Autodesk Inventor part; units mm, degrees
(part 2 of 2)
  spline S27 degree 3 poles (53.2343, -1.5147) (53.2876, -1.6132) (53.3942, -1.8104) (53.5388, -2.114) (53.6487, -2.3717) (53.7287, -2.5811) (53.7846, -2.7396) (53.8352, -2.8999) (53.8989, -3.1148) (53.9296, -3.3095) (53.9849, -3.4685) (54.0166, -3.5312) (54.0472, -3.5782) (54.0738, -3.6107) (54.1026, -3.6414) (54.1344, -3.6689) (54.1689, -3.6931) (54.2057, -3.7134) (54.2441, -3.7308) (54.2847, -3.7418) (54.3257, -3.7514) (54.3818, -3.7547) (54.4518, -3.7553) (54.5217, -3.7582) (54.5779, -3.7578) (54.6193, -3.7503) (54.6605, -3.7414) (54.6997, -3.726) (54.7375, -3.7075) (54.7732, -3.6852) (54.8063, -3.6593) (54.8366, -3.6301) (54.8649, -3.599) (54.8979, -3.5536) (54.9327, -3.4926) (54.996, -3.3366) (55.0366, -3.1438) (55.1111, -2.9324) (55.1699, -2.7749) (55.2338, -2.6194) (55.3243, -2.4144) (55.4472, -2.1626) (55.607, -1.8667) (55.7235, -1.6753) (55.7818, -1.5795) knots 0 0 0 0 0.033613 0.067227 0.100839 0.117647 0.134454 0.151261 0.168068 0.201677 0.210077 0.218473 0.222676 0.226878 0.231076 0.235279 0.239479 0.24368 0.247882 0.252083 0.256283 0.260485 0.268889 0.277292 0.281494 0.285694 0.289895 0.294097 0.298298 0.302498 0.306701 0.310899 0.315101 0.319304 0.3277 0.3361 0.369709 0.386516 0.403323 0.420131 0.436938 0.470551 0.504164 0.537777 0.537777 0.537777 0.537777 projected
  arc A27 (53.2343, -1.5147) -> (52.4787, -1.5579) centre (54, -21.5) ccw projected
  spline S28 degree 3 poles (49.9552, -1.9133) (50.024, -2.0017) (50.1616, -2.1786) (50.3542, -2.4543) (50.5051, -2.6904) (50.6184, -2.8838) (50.6997, -3.0309) (50.776, -3.1807) (50.8742, -3.3822) (50.9365, -3.5691) (51.0172, -3.7169) (51.0588, -3.7735) (51.0967, -3.8148) (51.1284, -3.8426) (51.1618, -3.8681) (51.1977, -3.89) (51.2357, -3.9081) (51.2753, -3.9222) (51.3161, -3.933) (51.358, -3.9371) (51.4, -3.9399) (51.4558, -3.9339) (51.525, -3.9229) (51.5944, -3.9143) (51.6498, -3.9047) (51.6894, -3.8904) (51.7285, -3.8749) (51.7647, -3.8533) (51.7989, -3.8288) (51.8304, -3.8009) (51.8588, -3.7699) (51.8839, -3.7362) (51.9067, -3.7008) (51.9317, -3.6506) (51.956, -3.5847) (51.9928, -3.4204) (52.0011, -3.2235) (52.0398, -3.0027) (52.0719, -2.8377) (52.1093, -2.6738) (52.1648, -2.4567) (52.2446, -2.1881) (52.3536, -1.87) (52.437, -1.662) (52.4787, -1.5579) knots 0 0 0 0 0.033613 0.067227 0.100839 0.117647 0.134454 0.151261 0.168068 0.201677 0.210077 0.218473 0.222676 0.226878 0.231076 0.235279 0.239479 0.24368 0.247882 0.252083 0.256283 0.260485 0.268889 0.277292 0.281494 0.285694 0.289895 0.294097 0.298298 0.302498 0.306701 0.310899 0.315101 0.319304 0.3277 0.3361 0.369709 0.386516 0.403323 0.420131 0.436938 0.470551 0.504164 0.537777 0.537777 0.537777 0.537777 projected
  arc A28 (49.9552, -1.9133) -> (49.2171, -2.0803) centre (54, -21.5) ccw projected
  spline S29 degree 3 poles (46.7865, -2.8462) (46.869, -2.9221) (47.0338, -3.0739) (47.2691, -3.3141) (47.4568, -3.5222) (47.6004, -3.6943) (47.7048, -3.8261) (47.8047, -3.9612) (47.9347, -4.1438) (48.027, -4.3179) (48.1309, -4.4504) (48.1812, -4.4994) (48.2254, -4.5339) (48.2612, -4.556) (48.2984, -4.5757) (48.3374, -4.5914) (48.3779, -4.603) (48.4193, -4.6104) (48.4612, -4.6144) (48.5032, -4.6115) (48.5451, -4.6073) (48.5992, -4.5922) (48.6656, -4.57) (48.7327, -4.5501) (48.7857, -4.5315) (48.8225, -4.5109) (48.8585, -4.4892) (48.8906, -4.4619) (48.9203, -4.4321) (48.9468, -4.3994) (48.9698, -4.3641) (48.989, -4.3267) (49.0056, -4.2881) (49.022, -4.2345) (49.0352, -4.1655) (49.0444, -3.9974) (49.0202, -3.8018) (49.022, -3.5776) (49.0264, -3.4096) (49.0364, -3.2418) (49.0554, -3.0185) (49.0899, -2.7404) (49.145, -2.4087) (49.1931, -2.1898) (49.2171, -2.0803) knots 0 0 0 0 0.033613 0.067227 0.100839 0.117647 0.134454 0.151261 0.168068 0.201677 0.210077 0.218473 0.222676 0.226878 0.231076 0.235279 0.239479 0.24368 0.247882 0.252083 0.256283 0.260485 0.268889 0.277292 0.281494 0.285694 0.289895 0.294097 0.298298 0.302498 0.306701 0.310899 0.315101 0.319304 0.3277 0.3361 0.369709 0.386516 0.403323 0.420131 0.436938 0.470551 0.504164 0.537777 0.537777 0.537777 0.537777 projected
  arc A29 (46.7865, -2.8462) -> (46.0859, -3.1324) centre (54, -21.5) ccw projected
  spline S30 degree 3 poles (43.8146, -4.2879) (43.9084, -4.3492) (44.096, -4.4718) (44.3676, -4.67) (44.587, -4.8444) (44.757, -4.9905) (44.8816, -5.1033) (45.0024, -5.2201) (45.1607, -5.3789) (45.2804, -5.5354) (45.4047, -5.6489) (45.4624, -5.689) (45.5117, -5.7157) (45.5506, -5.7317) (45.5905, -5.745) (45.6316, -5.7541) (45.6734, -5.7589) (45.7155, -5.7593) (45.7575, -5.7563) (45.7984, -5.7466) (45.8391, -5.7356) (45.89, -5.7117) (45.9518, -5.6789) (46.0147, -5.6483) (46.0639, -5.6212) (46.0968, -5.5948) (46.1287, -5.5675) (46.1559, -5.5352) (46.1803, -5.501) (46.2011, -5.4644) (46.2179, -5.4258) (46.2307, -5.3857) (46.2407, -5.3449) (46.2481, -5.2893) (46.2497, -5.2191) (46.2311, -5.0517) (46.1751, -4.8628) (46.14, -4.6414) (46.1167, -4.475) (46.0989, -4.3078) (46.0809, -4.0844) (46.0692, -3.8045) (46.0689, -3.4682) (46.0803, -3.2443) (46.0859, -3.1324) knots 0 0 0 0 0.033613 0.067227 0.100839 0.117647 0.134454 0.151261 0.168068 0.201677 0.210077 0.218473 0.222676 0.226878 0.231076 0.235279 0.239479 0.24368 0.247882 0.252083 0.256283 0.260485 0.268889 0.277292 0.281494 0.285694 0.289895 0.294097 0.298298 0.302498 0.306701 0.310899 0.315101 0.319304 0.3277 0.3361 0.369709 0.386516 0.403323 0.420131 0.436938 0.470551 0.504164 0.537777 0.537777 0.537777 0.537777 projected
  arc A30 (43.8146, -4.2879) -> (43.1707, -4.6856) centre (54, -21.5) ccw projected
  spline S31 degree 3 poles (41.1205, -6.1991) (41.2231, -6.2441) (41.4283, -6.3342) (41.7289, -6.485) (41.9739, -6.6209) (42.1656, -6.737) (42.3071, -6.8277) (42.4455, -6.9231) (42.6278, -7.0536) (42.7716, -7.1883) (42.9129, -7.2799) (42.9764, -7.3099) (43.0294, -7.3282) (43.0705, -7.3375) (43.112, -7.344) (43.154, -7.3462) (43.1961, -7.3441) (43.2376, -7.3375) (43.2786, -7.3277) (43.3174, -7.3114) (43.3556, -7.2938) (43.4019, -7.2619) (43.4575, -7.2194) (43.5145, -7.1788) (43.5586, -7.144) (43.5866, -7.1126) (43.6137, -7.0803) (43.6351, -7.0441) (43.6536, -7.0063) (43.668, -6.9667) (43.6783, -6.9259) (43.6843, -6.8843) (43.6875, -6.8424) (43.6856, -6.7863) (43.6757, -6.7168) (43.6298, -6.5548) (43.5434, -6.3777) (43.4723, -6.1651) (43.422, -6.0047) (43.3769, -5.8428) (43.3224, -5.6254) (43.2647, -5.3512) (43.2092, -5.0195) (43.1835, -4.7969) (43.1707, -4.6856) knots 0 0 0 0 0.033613 0.067227 0.100839 0.117647 0.134454 0.151261 0.168068 0.201677 0.210077 0.218473 0.222676 0.226878 0.231076 0.235279 0.239479 0.24368 0.247882 0.252083 0.256283 0.260485 0.268889 0.277292 0.281494 0.285694 0.289895 0.294097 0.298298 0.302498 0.306701 0.310899 0.315101 0.319304 0.3277 0.3361 0.369709 0.386516 0.403323 0.420131 0.436938 0.470551 0.504164 0.537777 0.537777 0.537777 0.537777 projected
  arc A31 (41.1205, -6.1991) -> (40.5508, -6.6973) centre (54, -21.5) ccw projected
  spline S32 degree 3 poles (38.7777, -8.5277) (38.8863, -8.5552) (39.1036, -8.6103) (39.4249, -8.7096) (39.6889, -8.8032) (39.8971, -8.8862) (40.0516, -8.9524) (40.2039, -9.0237) (40.4051, -9.1225) (40.5691, -9.2316) (40.7236, -9.2987) (40.7911, -9.3178) (40.8464, -9.3271) (40.8884, -9.3296) (40.9305, -9.3292) (40.9723, -9.3244) (41.0134, -9.3154) (41.0533, -9.3021) (41.0921, -9.2857) (41.1277, -9.2632) (41.1626, -9.2396) (41.2029, -9.2005) (41.2508, -9.1494) (41.3003, -9.1) (41.3381, -9.0584) (41.3606, -9.0228) (41.3819, -8.9865) (41.3971, -8.9472) (41.4091, -8.9069) (41.4169, -8.8655) (41.4203, -8.8236) (41.4194, -8.7815) (41.4156, -8.7396) (41.4045, -8.6847) (41.3832, -8.6177) (41.3113, -8.4655) (41.197, -8.305) (41.0919, -8.107) (41.0158, -7.9571) (40.9447, -7.8048) (40.8552, -7.5994) (40.7531, -7.3384) (40.6437, -7.0204) (40.5818, -6.805) (40.5508, -6.6973) knots 0 0 0 0 0.033613 0.067227 0.100839 0.117647 0.134454 0.151261 0.168068 0.201677 0.210077 0.218473 0.222676 0.226878 0.231076 0.235279 0.239479 0.24368 0.247882 0.252083 0.256283 0.260485 0.268889 0.277292 0.281494 0.285694 0.289895 0.294097 0.298298 0.302498 0.306701 0.310899 0.315101 0.319304 0.3277 0.3361 0.369709 0.386516 0.403323 0.420131 0.436938 0.470551 0.504164 0.537777 0.537777 0.537777 0.537777 projected
  arc A32 (38.7777, -8.5277) -> (38.2978, -9.1129) centre (54, -21.5) ccw projected
  spline S33 degree 3 poles (36.8501, -11.2101) (36.9618, -11.2194) (37.1852, -11.238) (37.5184, -11.283) (37.7943, -11.3319) (38.0133, -11.3795) (38.1766, -11.4194) (38.3385, -11.4646) (38.5533, -11.5289) (38.733, -11.6096) (38.8964, -11.6503) (38.9662, -11.6581) (39.0223, -11.6582) (39.0641, -11.6537) (39.1055, -11.6464) (39.146, -11.6348) (39.185, -11.6191) (39.2222, -11.5994) (39.2578, -11.5768) (39.2892, -11.5488) (39.3196, -11.5198) (39.353, -11.4746) (39.3918, -11.4163) (39.4326, -11.3594) (39.463, -11.3122) (39.4793, -11.2733) (39.4944, -11.2341) (39.5029, -11.1928) (39.5081, -11.1511) (39.5089, -11.109) (39.5054, -11.067) (39.4975, -11.0257) (39.4869, -10.985) (39.467, -10.9326) (39.4349, -10.8701) (39.339, -10.7318) (39.1998, -10.5923) (39.0635, -10.4143) (38.9638, -10.279) (38.8686, -10.1404) (38.7465, -9.9525) (38.6029, -9.7119) (38.4426, -9.4163) (38.3461, -9.214) (38.2978, -9.1129) knots 0 0 0 0 0.033613 0.067227 0.100839 0.117647 0.134454 0.151261 0.168068 0.201677 0.210077 0.218473 0.222676 0.226878 0.231076 0.235279 0.239479 0.24368 0.247882 0.252083 0.256283 0.260485 0.268889 0.277292 0.281494 0.285694 0.289895 0.294097 0.298298 0.302498 0.306701 0.310899 0.315101 0.319304 0.3277 0.3361 0.369709 0.386516 0.403323 0.420131 0.436938 0.470551 0.504164 0.537777 0.537777 0.537777 0.537777 projected
  arc A33 (36.8501, -11.2101) -> (36.4731, -11.8663) centre (54, -21.5) ccw projected
  spline S34 degree 3 poles (35.3904, -14.1732) (35.5021, -14.164) (35.7254, -14.1456) (36.0615, -14.1351) (36.3417, -14.138) (36.5656, -14.1488) (36.7332, -14.1613) (36.9003, -14.1793) (37.1227, -14.2074) (37.3133, -14.2574) (37.4812, -14.2706) (37.5513, -14.2668) (37.6066, -14.2576) (37.6471, -14.2463) (37.6868, -14.2323) (37.7248, -14.2142) (37.7607, -14.1923) (37.7942, -14.1668) (37.8255, -14.1387) (37.8519, -14.1058) (37.8772, -14.0722) (37.9027, -14.0221) (37.9313, -13.9583) (37.9622, -13.8954) (37.9844, -13.8438) (37.9941, -13.8029) (38.0025, -13.7616) (38.0041, -13.7195) (38.0024, -13.6775) (37.9962, -13.6358) (37.9859, -13.5951) (37.9713, -13.5556) (37.9541, -13.5172) (37.9259, -13.4688) (37.884, -13.4124) (37.7665, -13.2918) (37.6063, -13.1771) (37.4426, -13.0239) (37.322, -12.9069) (37.2053, -12.7859) (37.0539, -12.6207) (36.8726, -12.4069) (36.6659, -12.1417) (36.5374, -11.9581) (36.4731, -11.8663) knots 0 0 0 0 0.033613 0.067227 0.100839 0.117647 0.134454 0.151261 0.168068 0.201677 0.210077 0.218473 0.222676 0.226878 0.231076 0.235279 0.239479 0.24368 0.247882 0.252083 0.256283 0.260485 0.268889 0.277292 0.281494 0.285694 0.289895 0.294097 0.298298 0.302498 0.306701 0.310899 0.315101 0.319304 0.3277 0.3361 0.369709 0.386516 0.403323 0.420131 0.436938 0.470551 0.504164 0.537777 0.537777 0.537777 0.537777 projected
  arc A34 (35.3904, -14.1732) -> (35.1265, -14.8826) centre (54, -21.5) ccw projected
  spline S35 degree 3 poles (34.4382, -17.3362) (34.5469, -17.3087) (34.7642, -17.2538) (35.094, -17.1881) (35.3708, -17.1448) (35.5934, -17.1187) (35.7608, -17.1034) (35.9286, -17.0937) (36.1526, -17.0847) (36.3488, -17.1027) (36.5165, -17.0881) (36.5851, -17.0728) (36.6382, -17.0547) (36.6763, -17.0369) (36.7131, -17.0165) (36.7476, -16.9924) (36.7794, -16.9649) (36.8082, -16.9342) (36.8345, -16.9013) (36.8551, -16.8646) (36.8745, -16.8272) (36.8914, -16.7737) (36.9092, -16.7059) (36.9292, -16.6389) (36.9426, -16.5843) (36.9455, -16.5423) (36.947, -16.5003) (36.9416, -16.4585) (36.933, -16.4173) (36.9201, -16.3772) (36.9032, -16.3387) (36.8823, -16.3022) (36.8591, -16.2671) (36.8232, -16.224) (36.7726, -16.1753) (36.6369, -16.0757) (36.46, -15.9889) (36.2733, -15.8648) (36.1351, -15.7692) (36, -15.6691) (35.8235, -15.531) (35.6096, -15.35) (35.362, -15.1225) (35.205, -14.9625) (35.1265, -14.8826) knots 0 0 0 0 0.033613 0.067227 0.100839 0.117647 0.134454 0.151261 0.168068 0.201677 0.210077 0.218473 0.222676 0.226878 0.231076 0.235279 0.239479 0.24368 0.247882 0.252083 0.256283 0.260485 0.268889 0.277292 0.281494 0.285694 0.289895 0.294097 0.298298 0.302498 0.306701 0.310899 0.315101 0.319304 0.3277 0.3361 0.369709 0.386516 0.403323 0.420131 0.436938 0.470551 0.504164 0.537777 0.537777 0.537777 0.537777 projected
  arc A35 (34.4382, -17.3362) -> (34.2947, -18.0793) centre (54, -21.5) ccw projected
  spline S36 degree 3 poles (34.0197, -20.6127) (34.1223, -20.5677) (34.3276, -20.4778) (34.6421, -20.3588) (34.908, -20.2705) (35.1233, -20.2081) (35.2859, -20.1655) (35.4498, -20.1282) (35.6693, -20.0825) (35.8658, -20.068) (36.0288, -20.026) (36.0939, -19.9996) (36.1433, -19.973) (36.1779, -19.9491) (36.2109, -19.923) (36.2409, -19.8935) (36.2678, -19.8612) (36.2912, -19.8262) (36.3117, -19.7894) (36.3259, -19.7498) (36.3389, -19.7097) (36.3468, -19.6541) (36.3532, -19.5844) (36.3619, -19.5149) (36.3662, -19.4589) (36.3621, -19.417) (36.3566, -19.3753) (36.3445, -19.3349) (36.3292, -19.2958) (36.3099, -19.2584) (36.2868, -19.2232) (36.2603, -19.1905) (36.2315, -19.1598) (36.1891, -19.1232) (36.1311, -19.0835) (35.9809, -19.0075) (35.7921, -18.9511) (35.5875, -18.8594) (35.4355, -18.7878) (35.2858, -18.7113) (35.0889, -18.6042) (34.8481, -18.4609) (34.5665, -18.2772) (34.3853, -18.1452) (34.2947, -18.0793) knots 0 0 0 0 0.033613 0.067227 0.100839 0.117647 0.134454 0.151261 0.168068 0.201677 0.210077 0.218473 0.222676 0.226878 0.231076 0.235279 0.239479 0.24368 0.247882 0.252083 0.256283 0.260485 0.268889 0.277292 0.281494 0.285694 0.289895 0.294097 0.298298 0.302498 0.306701 0.310899 0.315101 0.319304 0.3277 0.3361 0.369709 0.386516 0.403323 0.420131 0.436938 0.470551 0.504164 0.537777 0.537777 0.537777 0.537777 projected
  arc A36 (34.0197, -20.6127) -> (34.0004, -21.3693) centre (54, -21.5) ccw projected
  spline S37 degree 3 poles (34.1462, -23.9135) (34.24, -23.8522) (34.4277, -23.7297) (34.7183, -23.5605) (34.9661, -23.4297) (35.1681, -23.3327) (35.3215, -23.2639) (35.477, -23.2002) (35.686, -23.119) (35.8774, -23.0723) (36.0313, -23.0041) (36.0912, -22.9673) (36.1355, -22.9329) (36.1657, -22.9037) (36.1939, -22.8725) (36.2187, -22.8385) (36.2399, -22.8021) (36.2572, -22.7638) (36.2714, -22.7241) (36.2789, -22.6827) (36.2851, -22.641) (36.2838, -22.5849) (36.2786, -22.5151) (36.2758, -22.4451) (36.2707, -22.3892) (36.2598, -22.3485) (36.2476, -22.3083) (36.2289, -22.2705) (36.2074, -22.2343) (36.1822, -22.2006) (36.1537, -22.1697) (36.1221, -22.1419) (36.0887, -22.1163) (36.0408, -22.0872) (35.9771, -22.0575) (35.8164, -22.0073) (35.6209, -21.9828) (35.404, -21.926) (35.2422, -21.8804) (35.082, -21.8296) (34.8702, -21.7563) (34.6091, -21.6546) (34.3011, -21.5198) (34.1006, -21.4195) (34.0004, -21.3693) knots 0 0 0 0 0.033613 0.067227 0.100839 0.117647 0.134454 0.151261 0.168068 0.201677 0.210077 0.218473 0.222676 0.226878 0.231076 0.235279 0.239479 0.24368 0.247882 0.252083 0.256283 0.260485 0.268889 0.277292 0.281494 0.285694 0.289895 0.294097 0.298298 0.302498 0.306701 0.310899 0.315101 0.319304 0.3277 0.3361 0.369709 0.386516 0.403323 0.420131 0.436938 0.470551 0.504164 0.537777 0.537777 0.537777 0.537777 projected
  arc A37 (34.1462, -23.9135) -> (34.2517, -24.6629) centre (54, -21.5) ccw projected
  circle A38 centre (54, -21.5) radius 16 projected
  line L0 (0, 0) -> (79, 0) projected
  line L1 (79, 0) -> (74, 0)
  line L2 (74, 0) -> (74, -8)
  line L3 (74, -8) -> (79, -8)
  line L4 (79, -8) -> (79, 0)
  line L5 (57.7417, -28) -> (79, -28) projected
  line L6 (79, -28) -> (75, -28)
  line L7 (75, -28) -> (75, -24)
  line L8 (75, -24) -> (79, -24)
  line L9 (79, -24) -> (79, -28)
  point P0 (-12, -28)
  point P1 (74, 0)
  point P2 (75, -28)
  dimension "d19" = 5
  dimension "d20" = 8
  dimension "d90" = 4
  dimension "d91" = 4
  constraints: 16 end point, 4 parallel, 2 horizontal, 2 perpendicular
  measures "d19" distance of L3.end L2.end
  measures "d20" distance of L2.end L1.end
  measures "d90" distance of L7.end L8.end
  measures "d91" distance of L6.end L7.end
extrude "forbackinsert" [suppressed]
sketch "Sketch6" plane through (12, 29.5, 0) normal (0, -1, 0) x (1, 0, 0)
  line L0 (74, 20) -> (74, 28) projected
  line L1 (0, 28) -> (74, 28) projected
  line L2 (0, 0) -> (0, 28) projected
  line L3 (0, 0) -> (20.9709, 0) projected
  arc A0 (27.6477, 0) -> (20.9709, 0) centre (24.3093, 2.2034) ccw projected
  line L4 (27.6477, 0) -> (50.2583, 0) projected
  arc A1 (57.7417, 0) -> (50.2583, 0) centre (54, 6.5) ccw projected
  line L5 (79, 4) -> (79, 20) projected
  line L6 (79, 20) -> (74, 20) projected
  circle A2 centre (13.5, 14) radius 7 projected
  line L7 (-32.5699, 5.3617) -> (-52.5639, 19.3617) projected
  line L8 (-51.4168, 23) -> (-36.5545, 23) projected
  line L9 (-35.4073, 22.6383) -> (-15.4133, 8.6383) projected
  line L10 (-16.5604, 5) -> (2.5, 5) projected
  line L11 (2.5, 5) -> (2.5, 20) projected
  line L12 (8.5, 26) -> (22.5, 26) projected
  line L13 (25, 22) -> (29, 22) projected
  line L14 (29, 22) -> (29, 28) projected
  line L15 (29, 28) -> (-65.4385, 28) projected
  line L16 (-65.4385, 28) -> (-87.1068, 12.8277) projected
  arc A3 (-87.5314, 10.9816) -> (-87.1068, 12.8277) centre (-98.9773, 14.5858) ccw projected
  line L17 (-87.5314, 10) -> (-87.5314, 10.9816) projected
  line L18 (-74.6, 10) -> (-87.5314, 10) projected
  line L19 (-74.6, 9.8773) -> (-74.6, 10) projected
  line L20 (-74.6, 9.8773) -> (-69.3941, 9.2842) projected
  line L21 (-69.3941, 9.2842) -> (-69.8116, 5.6194) projected
  line L22 (-69.8116, 5.6194) -> (-74.6, 6.165) projected
  line L23 (-74.6, 0) -> (-74.6, 6.165) projected
  line L24 (-74.6, 0) -> (-71.1217, 0) projected
  line L25 (-71.1217, 4) -> (-71.1217, 0) projected
  line L26 (-71.1217, 4) -> (-61.009, 4) projected
  line L27 (-61.009, 4) -> (-50.8963, 4) projected
  line L28 (-50.8963, 0) -> (-50.8963, 4) projected
  line L29 (-50.8963, 0) -> (-46.5247, 0) projected
  line L30 (-46.5247, 4) -> (-46.5247, 0) projected
  line L31 (-46.5247, 4) -> (-36.4119, 4) projected
  line L32 (-36.4119, 4) -> (-26.2992, 4) projected
  line L33 (-26.2992, 0) -> (-26.2992, 4) projected
  line L34 (-26.2992, 0) -> (-17.2172, 0) projected
  line L35 (-17.2172, 5) -> (-17.2172, 0) projected
  line L36 (-17.2172, 5) -> (-31.4227, 5) projected
  line L37 (-57.1669, 5.3617) -> (-69.8981, 14.2761) projected
  line L38 (-69.8981, 17.5527) -> (-65.445, 20.6708) projected
  line L39 (-63.1507, 20.6708) -> (-45.9666, 8.6383) projected
  line L40 (-4.6472, 7.2037) -> (-24.8669, 21.3617) projected
  line L41 (-23.7198, 25) -> (-3.5, 25) projected
  line L42 (-1.5, 23) -> (-1.5, 8.842) projected
  line L43 (29, 28) -> (23, 28)
  line L44 (23, 28) -> (23, 22)
  line L45 (23, 22) -> (29, 22)
  line L46 (29, 22) -> (29, 28)
  line L47 (79, 28) -> (0, 28) projected
  line L48 (0, 28) -> (6, 28)
  line L49 (6, 28) -> (6, 22)
  line L50 (6, 22) -> (0, 22)
  line L51 (0, 22) -> (0, 28)
  line L52 (6, 22) -> (24.3093, 2.2034) construction
  line L53 (24.3093, 2.2034) -> (39.5, 28) construction
  line L54 (39.5, 28) -> (54, 6.5) construction
  line L55 (54, 6.5) -> (79, 28) construction
  line L56 (0, 3) -> (79, 3)
  line L57 (79, 0) -> (79, 28) projected
  line L58 (74, 25) -> (0, 25)
  line L59 (3, 25) -> (3, 3)
  circle A4 centre (13.5, 14) radius 7
  circle A5 centre (13.5, 14) radius 7 projected
  circle A6 centre (13.5, 14) radius 9
  line L60 (22.8927, 5.9442) -> (5.2686, 25)
  line L61 (3, 23.0345) -> (20.6903, 3.9072)
  line L62 (24.8983, 6.1598) -> (35.9927, 25)
  line L63 (39.4742, 25) -> (27.4834, 4.6375)
  line L64 (39.586, 25.1899) -> (48.6476, 11.7537)
  line L65 (51.1348, 13.4311) -> (43.3325, 25)
  line L66 (58.5934, 12.4288) -> (73.2112, 25)
  line L67 (76.7399, 24.0779) -> (60.5496, 10.1542)
  line L68 (76, 28) -> (76, 0)
  circle A7 centre (26, 25) radius 1.8 projected
  line L69 (75, 0) -> (75, 4) projected
  line L70 (75, 4) -> (79, 4) projected
  line L71 (-47.1137, 5) -> (-56.0198, 5) projected
  line L72 (57.7417, 0) -> (75, 0) projected
  circle A8 centre (24.3093, 2.2034) radius 2 projected
  circle A9 centre (3, 25) radius 1.8 projected
  arc A10 (4.5, 22) -> (6.5, 24) centre (4.5, 24) ccw projected
  arc A11 (8.5, 26) -> (6.5, 24) centre (8.5, 24) ccw projected
  circle A12 centre (13.5, 14) radius 14 projected
  line L73 (0, 28) -> (0, 0)
  line L74 (6, 22) -> (0, 28)
  line L75 (6, 28) -> (0, 22)
  arc A13 (23, 25.6082) -> (22.5, 26) centre (13.5, 14) ccw projected
  line L76 (23, 25.6082) -> (23, 24) projected
  arc A14 (23, 24) -> (25, 22) centre (25, 24) ccw projected
  arc A15 (-51.4168, 23) -> (-52.5639, 19.3617) centre (-51.4168, 21) ccw projected
  arc A16 (-35.4073, 22.6383) -> (-36.5545, 23) centre (-36.5545, 21) ccw projected
  arc A17 (-16.5604, 5) -> (-15.4133, 8.6383) centre (-16.5604, 7) ccw projected
  arc A18 (4.5, 22) -> (2.5, 20) centre (4.5, 20) ccw projected
  arc A19 (-32.5699, 5.3617) -> (-31.4227, 5) centre (-31.4227, 7) ccw projected
  arc A20 (-57.1669, 5.3617) -> (-56.0198, 5) centre (-56.0198, 7) ccw projected
  arc A21 (-69.8981, 17.5527) -> (-69.8981, 14.2761) centre (-68.7509, 15.9144) ccw projected
  arc A22 (-63.1507, 20.6708) -> (-65.445, 20.6708) centre (-64.2979, 19.0325) ccw projected
  arc A23 (-47.1137, 5) -> (-45.9666, 8.6383) centre (-47.1137, 7) ccw projected
  arc A24 (-4.6472, 7.2037) -> (-1.5, 8.842) centre (-3.5, 8.842) ccw projected
  arc A25 (-23.7198, 25) -> (-24.8669, 21.3617) centre (-23.7198, 23) ccw projected
  arc A26 (-1.5, 23) -> (-3.5, 25) centre (-3.5, 23) ccw projected
  point P0 (-12, 0)
  point P1 (33.4788, 14.8188)
  point P2 (20.3894, 3)
  point P3 (3, 5)
  point P4 (3, 22)
  point P5 (3, 22)
  point P6 (3.9568, 22)
  point P7 (6.3276, 19.4366)
  point P8 (18.361, 6.4257)
  point P9 (20.5805, 8.4442)
  point P10 (8.513, 21.492)
  point P11 (6, 24.2092)
  point P12 (6, 25)
  point P13 (23, 25)
  point P14 (29, 22)
  point P15 (29, 25)
  point P16 (39.714, 25)
  point P17 (74, 21.7216)
  point P18 (47.3668, 3)
  point P19 (28.2292, 3)
  point P20 (76, 20)
  point P21 (76, 3)
  point P22 (60.6332, 3)
  point P23 (0, 5)
  point P24 (21, 20.6569)
  point P25 (21.4833, 20)
  point P26 (29, 22)
  point P27 (0, 22)
  point P28 (0, 25)
  point P29 (6, 28)
  point P30 (8, 26)
  point P31 (21, 26)
  point P32 (3, 5)
  point P33 (2.5, 20)
  point P34 (75, 3)
  point P35 (76, 4)
  point P36 (79, 4)
  point P37 (6.7918, 20)
  point P38 (3, 5)
  point P39 (0, 5)
  point P40 (8, 21.1239)
  point P41 (29, 25)
  point P42 (26.1438, 3)
  point P43 (22.4748, 3)
  point P44 (0, 24.005)
  point P45 (0, 25.995)
  point P46 (3, 23.2)
  point P47 (6.7679, 25)
  point P48 (2.5, 24)
  point P49 (-0.5, 14)
  point P50 (0, 14)
  point P51 (6, 25.9365)
  point P52 (3.632, 22.3512)
  point P53 (4.5, 22)
  point P54 (6, 22.6771)
  point P55 (6.4765, 23.694)
  point P56 (2.9479, 23.2008)
  point P57 (3, 23.2601)
  point P58 (4.8397, 25)
  point P59 (4.7997, 24.9684)
  point P60 (4.8, 25)
  point P61 (22.1603, 3)
  point P62 (24.9891, 22)
  point P63 (24.9891, 22)
  point P64 (26.5875, 9.0284)
  point P65 (4.0126, 21.9397)
  point P66 (4.5, 22)
  point P67 (22.1603, 25)
  point P68 (23, 24.2835)
  point P69 (22.9581, 3.678)
  dimension "d23" = 6
  dimension "d24" = 6
  dimension "d25" = 6
  dimension "d26" = 6
  dimension "d27" = 3
  dimension "d28" = 3
  dimension "d29" = 3
  dimension "d31" = 18
  dimension "d32" = 1.5
  dimension "d33" = 1.5
  dimension "d34" = 1.5
  dimension "d35" = 1.5
  dimension "d36" = 1.5
  dimension "d37" = 1.5
  dimension "d38" = 1.5
  dimension "d39" = 1.5
  dimension "d40" = 3
  dimension "d105" = 0.5
  constraints: 54 end point, 14 point on line, 13 parallel, 8 point on circle, 6 perpendicular, 4 midpoint, 3 coincident, 2 centre point, 2 horizontal, 2 other
  measures "d23" distance of L45.end L44.end
  measures "d24" distance of L44.end L43.end
  measures "d25" distance of L49.end L50.end
  measures "d26" distance of L48.end L49.end
  measures "d27" distance between parallel lines of L2 L59
  measures "d28" distance between parallel lines of L56 L3
  measures "d29" distance between parallel lines of L1 L58
  measures "d31" diameter of A6
  measures "d32" distance between parallel lines of L52 L61
  measures "d33" distance between parallel lines of L52 L60
  measures "d34" distance between parallel lines of L62 L53
  measures "d35" distance from line of L53 point (33.479, 14.819)
  measures "d36" distance between parallel lines of L64 L54
  measures "d37" distance between parallel lines of L54 L65
  measures "d38" distance between parallel lines of L55 L67
  measures "d39" distance between parallel lines of L55 L66
  measures "d40" distance between parallel lines of L68 L5
  measures "d105" distance of point (0, 14) point (-0.5, 14)
extrude "zeberka" [suppressed]
fillet "Fillet1" [suppressed]
fillet "Fillet2" [suppressed]
fillet "Fillet3" [suppressed]
ref_plane "Work Plane4" through (0, 0, 0) normal (0, 0, 1) x (1, 0, 0)
sketch "Sketch9" plane through (0, 0, 0) normal (0, 0, 1) x (1, 0, 0)
  line L0 (-71, -74) -> (-71, -89) projected
  line L1 (-71, -89) -> (41, -89) projected
  line L2 (41, -89) -> (41, -30.5) projected
  line L3 (41, -30.5) -> (91, -30.5) projected
  line L4 (91, -30.5) -> (91, -26.5) projected
  line L5 (91, 30.5) -> (41, 30.5) projected
  line L6 (41, 30.5) -> (41, 89) projected
  line L7 (41, 89) -> (-71, 89) projected
  line L8 (-71, 89) -> (-71, 74) projected
  line L9 (-71, 74) -> (-87, 74) projected
  line L10 (-87, 74) -> (-87, 89) projected
  line L11 (-87, 89) -> (-91, 89) projected
  line L12 (-91, 89) -> (-91, -89) projected
  line L13 (-91, -89) -> (-87, -89) projected
  line L14 (-87, -89) -> (-87, -74) projected
  line L15 (-87, -74) -> (-71, -74) projected
  line L16 (91, 26.5) -> (86, 26.5) projected
  line L17 (91, 30.5) -> (91, 26.5) projected
  line L18 (12, 30.5) -> (12, 27.5) projected
  line L19 (12, 27.5) -> (18.5, 27.5)
  line L20 (18.5, 27.5) -> (18.5, 21)
  line L21 (18.5, 21) -> (12, 21)
  line L22 (12, 21) -> (12, 27.5)
  line L23 (18.5, 27.5) -> (18.5, 30.5)
  line L24 (84.2679, 27.5) -> (12, 27.5) projected
  circle A0 centre (15.25, 24.25) radius 1.8 projected
  circle A1 centre (15.25, -15.75) radius 1.8 projected
  circle A2 centre (6.1414, -28.5) radius 1.8 projected
  circle A3 centre (-23.4, 24.1) radius 1.8 projected
  circle A4 centre (-71.6, -24.1) radius 1.8 projected
  circle A5 centre (-82.75, 33.75) radius 1.8 projected
  circle A6 centre (-67.5, -84.5) radius 1.8 projected
  circle A7 centre (88, -10.5) radius 1.8 projected
  circle A8 centre (88, 10.5) radius 1.8 projected
  circle A9 centre (-67.5, 84.5) radius 1.8 projected
  circle A10 centre (-71.6, 24.1) radius 1.8 projected
  circle A11 centre (-82.75, -33.75) radius 1.8 projected
  circle A12 centre (-23.4, -24.1) radius 1.8 projected
  circle A13 centre (15.25, -24.25) radius 1.8 projected
  circle A14 centre (15.25, 15.75) radius 1.8 projected
  circle A15 centre (6.1414, 28.5) radius 1.8 projected
  circle A16 centre (-51.4385, -83.5) radius 1.55 projected
  circle A17 centre (-24.4119, -29.75) radius 1.55 projected
  circle A18 centre (-49.009, 29.75) radius 1.55 projected
  circle A19 centre (-22.5, 83.5) radius 1.55 projected
  circle A20 centre (8.5, -82.4087) radius 1.55 projected
  circle A21 centre (8.5, 82.4087) radius 1.55 projected
  circle A22 centre (-51.4385, 83.5) radius 1.55 projected
  circle A23 centre (-24.4119, 29.75) radius 1.55 projected
  circle A24 centre (-49.009, -29.75) radius 1.55 projected
  circle A25 centre (-22.5, -83.5) radius 1.55 projected
  circle A26 centre (-83, 21.5) radius 1.8 projected
  circle A27 centre (-83, -64.5) radius 1.8 projected
  circle A28 centre (-83, -21.5) radius 1.8 projected
  circle A29 centre (-83, 64.5) radius 1.8 projected
  line L25 (91, 30.5) -> (12, 30.5) projected
  line L26 (12, 30.5) -> (12, 27.5) projected
  arc A30 (86, 26.5) -> (84.2679, 27.5) centre (84.2679, 25.5) ccw projected
  line L27 (87.7321, 26.5) -> (91, 26.5) projected
  line L28 (91, 26.5) -> (91, 30.5) projected
  line L29 (91, -26.5) -> (87.7321, -26.5) projected
  arc A31 (87.7321, -26.5) -> (86.866, -27) centre (87.7321, -27.5) ccw projected
  arc A32 (86, -27.5) -> (86.866, -27) centre (86, -26.5) ccw projected
  line L30 (86, -27.5) -> (41.8217, -27.5) projected
  ellipse E0 centre (41.4293, -27.1664) end of major axis (40.558, -26.9979) minor radius 0.2933 (41, -27.3523) -> (41.8217, -27.5) ccw projected
  line L31 (41, -27.3523) -> (41, -27.5) projected
  line L32 (41, -27.5) -> (18.5, -27.5) projected
  line L33 (18.5, -27.5) -> (18.5, -12.5) projected
  line L34 (18.5, -12.5) -> (91, -12.5) projected
  line L35 (91, -12.5) -> (91, 12.5) projected
  line L36 (91, 12.5) -> (18.5, 12.5) projected
  line L37 (18.5, 12.5) -> (18.5, 27.5) projected
  line L38 (18.5, 27.5) -> (41, 27.5) projected
  line L39 (41, 27.5) -> (41, 27.3523) projected
  ellipse E1 centre (41.4293, 27.1664) end of major axis (40.558, 26.9979) minor radius 0.2933 (41.8217, 27.5) -> (41, 27.3523) ccw projected
  line L40 (41.8217, 27.5) -> (86, 27.5) projected
  arc A33 (86.866, 27) -> (86, 27.5) centre (86, 26.5) ccw projected
  arc A34 (86.866, 27) -> (87.7321, 26.5) centre (87.7321, 27.5) ccw projected
  line L41 (-85, 14) -> (-76, 14) projected
  line L42 (-76, 14) -> (-76, 20.1) projected
  line L43 (-76, 20.1) -> (11.5, 20.1) projected
  line L44 (11.5, 20.1) -> (11.5, 8.5) projected
  line L45 (11.5, 8.5) -> (84, 8.5) projected
  line L46 (84, 8.5) -> (84, -8.5) projected
  line L47 (84, -8.5) -> (11.5, -8.5) projected
  line L48 (11.5, -8.5) -> (11.5, -20.1) projected
  line L49 (11.5, -20.1) -> (-76, -20.1) projected
  line L50 (-76, -20.1) -> (-76, -14) projected
  line L51 (-76, -14) -> (-85, -14) projected
  arc A35 (-87, -12) -> (-85, -14) centre (-85, -12) ccw projected
  line L52 (-87, -12) -> (-87, 12) projected
  arc A36 (-85, 14) -> (-87, 12) centre (-85, 12) ccw projected
  line L53 (-76, 57) -> (-64, 69) projected
  line L54 (-64, 69) -> (-64, 79.9087) projected
  line L55 (-64, 79.9087) -> (15.1148, 79.9087) projected
  line L56 (15.1148, 79.9087) -> (15.1148, 37) projected
  line L57 (15.1148, 37) -> (-86, 37) projected
  line L58 (-86, 37) -> (-86, 29.2679) projected
  arc A37 (-87, 31) -> (-86, 29.2679) centre (-85, 31) ccw projected
  line L59 (-87, 31) -> (-87, 55) projected
  arc A38 (-85, 57) -> (-87, 55) centre (-85, 55) ccw projected
  line L60 (-85, 57) -> (-76, 57) projected
  line L61 (-64, -79.9087) -> (-64, -69) projected
  line L62 (-64, -69) -> (-76, -57) projected
  line L63 (-76, -57) -> (-85, -57) projected
  arc A39 (-87, -55) -> (-85, -57) centre (-85, -55) ccw projected
  line L64 (-87, -55) -> (-87, -37) projected
  line L65 (-87, -37) -> (15.1148, -37) projected
  line L66 (15.1148, -37) -> (15.1148, -79.9087) projected
  line L67 (15.1148, -79.9087) -> (-64, -79.9087) projected
  line L68 (30.8852, 37) -> (20.1148, 37) projected
  line L69 (20.1148, 37) -> (20.1148, 79.9087) projected
  line L70 (20.1148, 79.9087) -> (30.8852, 79.9087) projected
  line L71 (30.8852, 79.9087) -> (30.8852, 37) projected
  line L72 (30.8852, -79.9087) -> (20.1148, -79.9087) projected
  line L73 (20.1148, -79.9087) -> (20.1148, -37) projected
  line L74 (20.1148, -37) -> (30.8852, -37) projected
  line L75 (30.8852, -37) -> (30.8852, -79.9087) projected
  point P0 (0, 0)
  point P1 (12, 29.5)
  dimension "d55" = 6.5
  dimension "d56" = 6.5
  constraints: 10 end point, 2 parallel, 1 horizontal, 1 perpendicular, 2 other
  measures "d55" distance of L20.end L21.end
  measures "d56" distance of L19.end L20.end
extrude "Extrusion6" add sketch "Sketch9" along normal blind 10 contours L23 L19 L18 L25 | L20 L21 L22 L19 | A0
fillet "Fillet4" [suppressed]
sketch "Sketch10" plane through (0, 0, 10) normal (0, 0, 1) x (1, 0, 0)
  line L0 (12, 21) -> (18.5, 21) projected
  line L1 (18.5, 21) -> (18.5, 27.5) projected
  line L2 (12, 27.5) -> (18.5, 21)
  line L3 (12, 27.5) -> (17, 27.5) projected
  line L4 (17.4377, 27.5) -> (18.5, 27.5) projected
  line L5 (12, 27.5) -> (12, 21) projected
  line L6 (17, 27.5) -> (17, 29.2956) projected
  line L7 (17.4377, 28.5) -> (17.4377, 27.5) projected
  point P0 (0, 0)
  point P1 (15.25, 24.25)
  constraints: 2 end point, 1 midpoint, 1 other
hole "Hole2" [suppressed]
sketch "Sketch11" plane through (0, 0, 28) normal (0, 0, 1) x (1, 0, 0)
  line L0 (49.9772, 27.5) -> (53.3587, 27.5)
  line L1 (49.9772, 27.5) -> (53.3587, 27.5)
  line L2 (34.4748, 27.5) -> (38.1438, 27.5)
  line L3 (49.9772, 27.5) -> (53.3587, 27.5)
  line L4 (91, 30.5) -> (12, 30.5)
  line L5 (49.6679, 30.5) -> (53.6679, 30.5)
  line L6 (53.6679, 30.5) -> (53.6679, 26.5)
  line L7 (53.6679, 26.5) -> (49.6679, 26.5)
  line L8 (49.6679, 26.5) -> (49.6679, 30.5)
  point P0 (0, 0)
  point P1 (56.6192, 27.5)
  point P2 (42.52, 28.5348)
  point P3 (53.3587, 29.5)
  point P4 (51.6679, 27.5)
  point P5 (51.6679, 27.5)
  point P6 (51.6679, 27.5)
  point P7 (53.6679, 30.5)
  point P8 (20.5, 27.5)
  point P9 (53.3587, 30.5)
  dimension "d67" = 1.6908
  dimension "d68" = 1.6908
  dimension "d69" = 4
  dimension "d70" = 4
  dimension "d71" = 2
  dimension "d72" = 2
  constraints: 14 end point, 2 coincident, 2 midpoint, 1 point on line, 7 other
  measures "d67" distance of L0.start point (51.668, 27.5)
  measures "d68" distance of point (51.668, 27.5) L0.end
  measures "d69" distance of L6.end L7.end
  measures "d70" distance of L5.end L6.end
  measures "d71" distance from line of point (51.668, 27.5) L6
  measures "d72" distance from line of L8 point (51.668, 27.5)
extrude "Extrusion7" add sketch "Sketch11" against normal blind 4
fillet "Fillet5" radius 1 1 edges at (51.6679, 26.5, 24)
sketch "Sketch12" plane through (0, 0, 28) normal (0, 0, 1) x (1, 0, 0)
  line L0 (49.6679, 26.5) -> (53.6679, 26.5) projected
  line L1 (53.6679, 26.5) -> (49.6679, 26.5)
  line L2 (49.6679, 26.5) -> (49.6679, 30.5)
  line L3 (49.6679, 30.5) -> (53.6679, 30.5)
  line L4 (53.6679, 30.5) -> (53.6679, 26.5)
  line L5 (49.6679, 26.5) -> (53.6679, 30.5)
  line L6 (49.6679, 30.5) -> (53.6679, 26.5)
  line L7 (53.6679, 27.5) -> (86, 27.5) projected
  arc A0 (86.866, 27) -> (86, 27.5) centre (86, 26.5) ccw projected
  arc A1 (86.866, 27) -> (87.7321, 26.5) centre (87.7321, 27.5) ccw projected
  line L8 (87.7321, 26.5) -> (91, 26.5) projected
  line L9 (91, 26.5) -> (91, 30.5) projected
  line L10 (91, 30.5) -> (41, 30.5) projected
  line L11 (41, 30.5) -> (41, 89) projected
  line L12 (41, 89) -> (-71, 89) projected
  line L13 (-71, 89) -> (-71, 74) projected
  line L14 (-71, 74) -> (-87, 74) projected
  line L15 (-87, 74) -> (-87, 89) projected
  line L16 (-87, 89) -> (-91, 89) projected
  line L17 (-91, 89) -> (-91, -89) projected
  line L18 (-91, -89) -> (-87, -89) projected
  line L19 (-87, -89) -> (-87, -74) projected
  line L20 (-87, -74) -> (-71, -74) projected
  line L21 (-71, -74) -> (-71, -89) projected
  line L22 (-71, -89) -> (41, -89) projected
  line L23 (41, -89) -> (41, -30.5) projected
  line L24 (41, -30.5) -> (91, -30.5) projected
  line L25 (91, -30.5) -> (91, -26.5) projected
  line L26 (91, -26.5) -> (87.7321, -26.5) projected
  arc A2 (87.7321, -26.5) -> (86.866, -27) centre (87.7321, -27.5) ccw projected
  arc A3 (86, -27.5) -> (86.866, -27) centre (86, -26.5) ccw projected
  line L27 (86, -27.5) -> (41.8217, -27.5) projected
  ellipse E0 centre (41.4293, -27.1664) end of major axis (42.3006, -27.3349) minor radius 0.2933 (41, -27.3523) -> (41.8217, -27.5) ccw projected
  line L28 (41, -27.3523) -> (41, -27.5) projected
  line L29 (41, -27.5) -> (18.5, -27.5) projected
  line L30 (18.5, -27.5) -> (18.5, -12.5) projected
  line L31 (18.5, -12.5) -> (91, -12.5) projected
  line L32 (91, -12.5) -> (91, 12.5) projected
  line L33 (91, 12.5) -> (18.5, 12.5) projected
  line L34 (18.5, 12.5) -> (18.5, 27.5) projected
  line L35 (18.5, 27.5) -> (41, 27.5) projected
  line L36 (41, 27.5) -> (41, 27.3523) projected
  ellipse E1 centre (41.4293, 27.1664) end of major axis (42.3006, 27.3349) minor radius 0.2933 (41.8217, 27.5) -> (41, 27.3523) ccw projected
  line L37 (41.8217, 27.5) -> (49.6679, 27.5) projected
  line L38 (49.6679, 27.5) -> (49.6679, 26.5) projected
  line L39 (53.6679, 26.5) -> (53.6679, 27.5) projected
  point P0 (0, 0)
  point P1 (51.6679, 28.5)
  constraints: 12 end point, 2 parallel, 2 perpendicular, 1 horizontal, 1 midpoint, 2 other
hole "Hole3" at (51.6679, 28.5, 28) direction (0, 0, -1) diameter 3 depth 3 counterbore diameter 3.5 counterbore depth 1
sketch "Sketch13" plane through (12, 27.5, 0) normal (0, -1, 0) x (1, 0, 0)
  circle A0 centre (26, 25) radius 1.8 projected
  circle A1 centre (3, 25) radius 1.8 projected
  point P0 (-12, 0)
  constraints: 3 coincident
hole "Hole4" [suppressed]
fillet "Fillet6" [suppressed]
sketch "Sketch14" plane through (91, 30.5, 28) normal (1, 0, 0) x (0, 0, -1)
  line L0 (28, -4) -> (24.7321, -4) projected
  line L1 (28, 0) -> (28, -4) projected
  line L2 (0, 0) -> (0, -4) projected
  line L3 (7.496, -4) -> (0, -4) projected
  line L4 (0, -4) -> (6, -4)
  line L5 (6, -4) -> (6, 0)
  line L6 (6, 0) -> (0, 0)
  line L7 (0, 0) -> (0, -4)
  line L8 (28, 0) -> (24, 0)
  line L9 (24, 0) -> (24, -4)
  line L10 (24, -4) -> (28, -4)
  line L11 (28, -4) -> (28, 0)
  line L12 (0, 0) -> (6, -4)
  line L13 (0, -4) -> (6, 0)
  line L14 (24, 0) -> (28, -4)
  line L15 (28, 0) -> (24, -4)
  line L16 (23, -3) -> (9.7321, -3) projected
  line L17 (28, 0) -> (0, 0) projected
  arc A0 (23.866, -3.5) -> (24.7321, -4) centre (24.7321, -3) ccw projected
  arc A1 (7.496, -4) -> (8.2413, -3.6667) centre (7.496, -3) ccw projected
  arc A2 (9.7321, -3) -> (8.2413, -3.6667) centre (9.7321, -5) ccw projected
  arc A3 (23.866, -3.5) -> (23, -3) centre (23, -4) ccw projected
  point P0 (28, -30.5)
  point P1 (26, -2)
  point P2 (3, -2)
  dimension "d93" = 6
  dimension "d94" = 4
  dimension "d95" = 4
  dimension "d96" = 4
  constraints: 24 end point, 4 parallel, 3 midpoint, 2 horizontal, 2 perpendicular
  measures "d93" distance of L6.end L5.end
  measures "d94" distance of L5.end L4.end
  measures "d95" distance of L10.end L9.end
  measures "d96" distance of L9.end L8.end
hole "Hole5" at (91, 28.5, 2) at (91, 28.5, 25) direction (-1, 0, 0) diameter 3 depth 3.5 counterbore diameter 3.5 counterbore depth 1
fillet "Fillet7" [suppressed]
sketch "Sketch15" plane through (36.3093, 26, 2.2034) normal (0, -1, 0) x (1, 0, 0)
  arc A0 (20.8931, 0.8835) -> (22.8499, -2.2034) centre (29.6907, 4.2966) ccw projected
  arc A1 (20.3099, 0.7966) -> (20.8931, 0.8835) centre (20.3099, 2.7966) ccw projected
  line L0 (20.3099, 0.7966) -> (5.8828, 0.7966) projected
  arc A2 (5.5124, -2.2034) -> (5.8828, 0.7966) centre (0, 0) ccw projected
  line L1 (5.5124, -2.2034) -> (22.8499, -2.2034) projected
  line L2 (54.6907, -2.2034) -> (-24.3093, -2.2034) projected
  line L3 (54.6907, -2.2034) -> (54.6907, 25.7966) projected
  line L4 (-24.3093, -2.2034) -> (54.6907, -2.2034)
  line L5 (-24.3093, -2.2034) -> (54.6907, -2.2034)
  line L6 (54.6907, -2.2034) -> (54.6907, -9.8273)
  line L7 (54.6907, -9.8273) -> (-24.3093, -9.8273)
  line L8 (-24.3093, -9.8273) -> (-24.3093, -2.2034)
  point P0 (-36.3093, -2.2034)
  point P1 (54.6907, -2.2034)
  constraints: 10 end point, 2 parallel, 1 horizontal, 1 perpendicular
extrude "Extrusion8" [suppressed]
equation "\"d33\" = d32"
equation "\"d34\" = d33"
equation "\"d35\" = d34"
equation "\"d36\" = d34"
equation "\"d37\" = d36"
equation "\"d38\" = d36"
equation "\"d39\" = d37"
body "Solid1"
